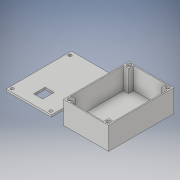
# Autodesk Inventor part: Box
Saved by Autodesk Inventor 2019 (Build 230136000, 136)
## iProperties
Created: 2018-08-26
Part Number: Box
Material: Generic
Document SubType Name: Modeling
Designer: a
Density: 1 g/cm^3
Appearance: Default
Author: a
Autodesk Inventor part; units mm, degrees
ref_plane "YZ Plane" through (0, 0, 0) normal (1, 0, 0) x (0, 1, 0)
ref_plane "XZ Plane" through (0, 0, 0) normal (0, 1, 0) x (-1, 0, 0)
ref_plane "XY Plane" through (0, 0, 0) normal (0, 0, 1) x (1, 0, 0)
sketch "Sketch1" plane through (0, 0, 0) normal (0, 1, 0) x (-1, 0, 0)
  line L0 (0, 0) -> (90, 0)
  line L1 (90, 0) -> (90, -130)
  line L2 (90, -130) -> (0, -130)
  line L3 (0, -130) -> (0, 0)
  dimension "d0" = 90
  dimension "d1" = 130
  constraints: 8 end point, 2 parallel, 1 horizontal, 1 perpendicular
  measures "d0" distance of L1.end L2.end
  measures "d1" distance of L0.end L1.end
extrude "Extrusion1" add sketch "Sketch1" along normal blind 45
shell "Shell1" thickness 2 removed faces 1 at (-30, 45, -43.3333)
sketch "Sketch2" plane through (-88, 2, -2) normal (0, 1, 0) x (1, 0, 0)
  line L0 (0, 0) -> (0, 126) projected
  line L1 (0, 0) -> (10, 0)
  line L2 (10, 0) -> (10, 10)
  line L3 (10, 10) -> (0, 10)
  line L4 (0, 10) -> (0, 0)
  point P0 (88, -2)
  dimension "d5" = 10
  dimension "d6" = 10
  constraints: 8 end point, 2 parallel, 1 horizontal, 1 perpendicular
  measures "d5" distance of L3.end L2.end
  measures "d6" distance of L2.end L1.end
extrude "Extrusion2" add sketch "Sketch2" along normal blind 43
pattern_linear "Rectangular Pattern1" count 2 spacing 116 along (0, 0, -1) count 2 spacing 76 along (1, 0, 0) of "Extrusion2"
sketch "Sketch3" plane through (0, 45, 0) normal (0, 1, 0) x (1, 0, 0)
  circle A0 centre (-6.5262, 6.3373) radius 4
  point P0 (0, 0)
  dimension "d15" = 8
  constraints: 1 centre point
  measures "d15" diameter of A0
extrude "Extrusion3" cut sketch "Sketch3" against normal blind 4
pattern_linear "Rectangular Pattern2" count 2 spacing 118 along (0, 0, -1) count 2 spacing 77 along (-1, 0, 0) of "Extrusion3"
sketch "Sketch4" plane through (-88, 2, -12) normal (0, 1, 0) x (1, 0, 0)
  line L0 (-25.9277, -12) -> (-115.9277, -12)
  line L1 (-115.9277, -12) -> (-115.9277, 118)
  line L2 (-115.9277, 118) -> (-25.9277, 118)
  line L3 (-25.9277, 118) -> (-25.9277, -12)
  point P0 (88, -12)
  dimension "d24" = 90
  dimension "d25" = 130
  constraints: 8 end point, 2 parallel, 1 horizontal, 1 perpendicular
  measures "d24" distance of L1.end L2.end
  measures "d25" distance of L0.end L1.end
extrude "Extrusion4" add sketch "Sketch4" along normal blind 4
sketch "Sketch5" plane through (-88, 6, -12) normal (0, 1, 0) x (1, 0, 0)
  circle A0 centre (-33.1465, -5.6627) radius 3.0421
  point P0 (88, -12)
  constraints: 1 centre point
extrude "Extrusion5" cut sketch "Sketch5" against normal blind 4
pattern_linear "Rectangular Pattern3" count 2 spacing 115 along (0, 0, -1) count 2 spacing 77 along (-1, 0, 0) of "Extrusion5"
sketch "Sketch6" plane through (-88, 6, -12) normal (0, 1, 0) x (1, 0, 0)
  line L0 (-70.9277, 6.57) -> (-79.9277, 6.57)
  line L1 (-79.9277, 6.57) -> (-79.9277, 29.57)
  line L2 (-79.9277, 29.57) -> (-61.9277, 29.57)
  line L3 (-61.9277, 29.57) -> (-61.9277, 6.57)
  line L4 (-61.9277, 6.57) -> (-70.9277, 6.57)
  point P0 (88, -12)
  dimension "d36" = 9
  dimension "d37" = 23
  dimension "d38" = 18
  constraints: 10 end point, 4 perpendicular, 1 horizontal, 1 point on line
  measures "d36" distance of L0.start L0.end
  measures "d37" distance of L0.end L1.end
  measures "d38" distance of L1.end L2.end
extrude "Extrusion6" cut sketch "Sketch6" against normal blind 4
body "Solid1"
